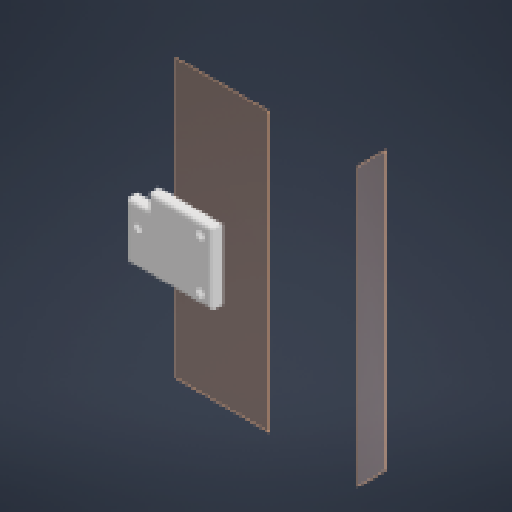
# Autodesk Inventor part: Print-head_Mount
Saved by Autodesk Inventor 2027.1 (Build 311270010, 270A)
## iProperties
Created: 2026-09-09
Part Number: Print-head_Mount
Material: Generic
Document SubType Name: Modeling
Designer: Jacob Parker
Density: 1 g/cm^3
Appearance: Default
Author: Jacob Parker
Autodesk Inventor part; units mm, degrees
ref_plane "YZ Plane" through (0, 0, 0) normal (1, 0, 0) x (0, 1, 0)
ref_plane "XZ Plane" through (0, 0, 0) normal (0, 1, 0) x (-1, 0, 0)
ref_plane "XY Plane" through (0, 0, 0) normal (0, 0, 1) x (1, 0, 0)
ref_plane "Work Plane1" through (55, -70.0761, -12.5) normal (1, 0, 0) x (0, 0, -1)
ref_plane "Work Plane2" through (-33.6954, 10.9239, 2.7231) normal (0, 0, 1) x (1, 0, 0)
sketch "Sketch2" plane through (-33.6954, 10.9239, 2.7231) normal (0, 0, 1) x (1, 0, 0)
  line L0 (-55, -33.4239) -> (0, -33.4239)
  line L1 (0, -33.4239) -> (0, 11.5761)
  line L2 (0, 11.5761) -> (-55, 11.5761)
  line L3 (-55, 11.5761) -> (-55, -33.4239)
  line L4 (-55, 1.5761) -> (-41, 1.5761)
  line L5 (-41, 1.5761) -> (-41, 11.5761)
  line L6 (-7.5, -26.9239) -> (-7.5, -33.4239)
  line L7 (-7.5, 5.0761) -> (-7.5, 11.5761)
  line L8 (-7.5, -26.9239) -> (0, -26.9239)
  line L9 (-47.5, -10.9239) -> (-55, -10.9239)
  point P0 (-27.5, 11.5761)
  dimension "d4" = 55
  dimension "d5" = 45
  dimension "d10" = 14
  dimension "d11" = 10
  dimension "d14" = 40
  dimension "d15" = 32
  dimension "d23" = 16
  constraints: 20 end point, 6 point on line, 5 equal length, 5 perpendicular, 2 horizontal, 2 midpoint, 1 other
  measures "d4" distance of L2.end L1.end
  measures "d5" distance of L2.end L0.start
  measures "d10" distance of L4.start L4.end
  measures "d11" distance of L4.end L5.end
  measures "d14" horizontal distance of L9.start L7.start
  measures "d15" distance of L7.start L6.start
  measures "d23" vertical distance of L9.start L7.start
extrude "Extrusion1" add sketch "Sketch2" along normal blind 7 contours L3 L4 L5 L2 L1 L8 L6 L0 | L6 L8 L1 L0
hole "Hole1" at (-41.1954, -16, 2.7231) at (-41.1954, 16, 2.7231) at (-81.1954, 0, 2.7231) direction (0, 0, 1) diameter 5 end through all
fillet "Fillet1" radius 2 6 edges at (-81.6954, 12.5, 9.7231) (-88.6954, -5, 9.7231) (-74.6954, 17.5, 9.7231) (-54.1954, 22.5, 9.7231) (-61.1954, -22.5, 9.7231) (-33.6954, 0, 9.7231)
body "Solid1"
